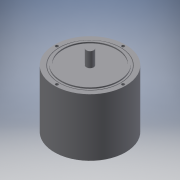
# Autodesk Inventor part: Denzel4500Motor
Saved by Autodesk Inventor 2018 (Build 220112000, 112)
## iProperties
Created: 2018-10-10
Part Number: Denzel4500Motor
Material: Generic
Document SubType Name: Modeling
Designer: eroldan
Density: 1 g/cm^3
Appearance: Default
Author: eroldan
Autodesk Inventor part; units mm, degrees
ref_plane "YZ Plane" through (0, 0, 0) normal (1, 0, 0) x (0, 1, 0)
ref_plane "XZ Plane" through (0, 0, 0) normal (0, 1, 0) x (-1, 0, 0)
ref_plane "XY Plane" through (0, 0, 0) normal (0, 0, 1) x (1, 0, 0)
sketch "Sketch1" plane through (0, 0, 0) normal (0, 0, 1) x (1, 0, 0)
  circle A0 centre (0, 0) radius 72.5
  dimension "d0" = 145
  constraints: 1 centre point, 1 coincident
  measures "d0" diameter of A0
extrude "Extrusion1" add sketch "Sketch1" along normal blind 120
sketch "Sketch2" plane through (0, 0, 120) normal (0, 0, 1) x (1, 0, 0)
  circle A0 centre (0, 0) radius 59
  circle A1 centre (0, 0) radius 54.75
  circle A2 centre (0, 0) radius 72.5 projected
  dimension "d3" = 118
  dimension "d4" = 109.5
  constraints: 2 centre point, 2 coincident
  measures "d3" diameter of A0
  measures "d4" diameter of A1
extrude "Extrusion2" cut sketch "Sketch2" against normal blind 2.5
sketch "Sketch3" plane through (0, 0, 117.5) normal (0, 0, 1) x (1, 0, 0)
  circle A0 centre (0, 0) radius 7.5
  dimension "d7" = 15
  constraints: 1 centre point, 1 coincident
  measures "d7" diameter of A0
extrude "Extrusion3" add sketch "Sketch3" along normal blind 30
sketch "Sketch4" plane through (0, 0, 117.5) normal (0, 0, 1) x (1, 0, 0)
  point P0 (0, 0)
  point P1 (0, 67.5)
  dimension "d10" = 67.5
  measures "d10" distance of point (0, 0) point (0, 67.5)
hole "Hole1" at (0, 67.5, 117.5) direction (0, 0, -1) diameter 6 end through all
pattern_circular "Circular Pattern1" count 4 over 360 about axis through (0, 0, 117.5) along (0, 0, 1) of "Hole1"
sketch "Sketch5" plane through (0, 0, 117.5) normal (0, 0, 1) x (1, 0, 0)
  circle A0 centre (0, 0) radius 62
  circle A1 centre (0, 0) radius 63
  dimension "d21" = 124
  dimension "d22" = 1
  constraints: 2 centre point, 1 coincident
  measures "d21" diameter of A0
  measures "d22" radial gap between concentric circles of A0 A1
extrude "Extrusion4" cut sketch "Sketch5" against normal through all
body "Solid1"
